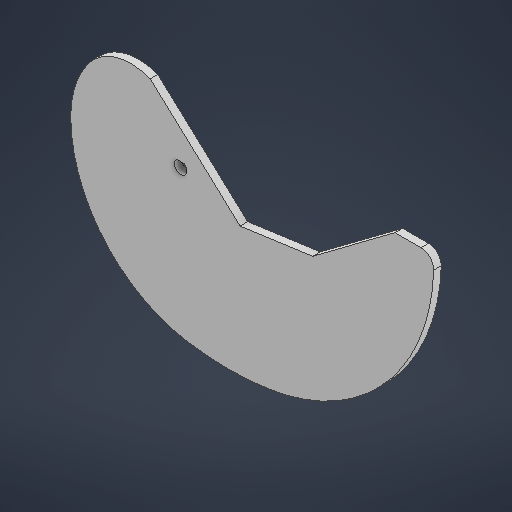
# Autodesk Inventor part: cam3
Saved by Autodesk Inventor 2027 (Build 310192000, 192)
## iProperties
Created: 2026-05-11
Part Number: cam3
Material: Generic
Document SubType Name: Modeling
Designer: alexy
Density: 1 g/cm^3
Appearance: Default
Mass: 17.9661 g
Surface Area: 129.636 cm^2
Volume: 17.9661 cm^3
Author: alexy
Autodesk Inventor part; units mm, degrees
ref_plane "YZ Plane" through (0, 0, 0) normal (1, 0, 0) x (0, 1, 0)
ref_plane "XZ Plane" through (0, 0, 0) normal (0, 1, 0) x (-1, 0, 0)
ref_plane "XY Plane" through (0, 0, 0) normal (0, 0, 1) x (1, 0, 0)
sketch "Sketch1" plane through (0, 0, 0) normal (0, 0, 1) x (1, 0, 0)
  line L0 (0, 0) -> (100, 0)
  arc A0 (100.0128, -3.6299) -> (100, 0) centre (-17.3055, -2.2293) ccw
  arc A1 (35.4459, -78.2987) -> (100.0128, -3.6299) centre (23.4974, -2.7164) ccw
  arc A2 (2.3748, -78.2085) -> (35.4459, -78.2987) centre (19.1908, 24.5253) ccw
  arc A3 (-43.4089, -24.3214) -> (2.3748, -78.2085) centre (11.1953, -24.3214) ccw
  arc A4 (-37.0013, -3.4804) -> (-43.4089, -24.3214) centre (-6.3121, -24.3214) ccw
  line L1 (84.6864, 0) -> (52.1966, -24.3214)
  line L2 (52.1966, -24.3214) -> (23.4974, -28.3171)
  line L3 (23.4974, -28.3171) -> (-12.0135, 4.2661)
  arc A5 (-12.0135, 4.2661) -> (-37.0013, -3.4804) centre (-19.6547, -15.2605) ccw
  point P0 (3.9425, 17.9592)
  dimension "d14" = 100
  constraints: 12 point on circle, 8 end point, 6 centre point, 5 tangent, 1 horizontal, 1 point on line
  measures "d14" distance of L0.start L0.end
extrude "Extrusion1" add sketch "Sketch1" along normal blind 3
sketch "Sketch2" plane through (0, 0, 3) normal (0, 0, 1) x (1, 0, 0)
  arc A0 (-1.5, -18) -> (1.5, -18) centre (0, -20) ccw
  line L0 (-1.5, -18) -> (1.5, -18)
  point P0 (0, 0)
  dimension "d5" = 5
  dimension "d6" = 20
  dimension "d7" = 2
  constraints: 2 end point, 2 point on circle, 1 centre point, 1 horizontal, 1 vertical alignment
  measures "d5" diameter of A0
  measures "d6" distance of point (0, 0) A0.centre
  measures "d7" distance from line of L0 A0.centre
extrude "Extrusion2" cut sketch "Sketch2" against normal blind 3
fillet "Fillet7" radius 5 1 edges at (100, 0, 1.5)
body "Solid1"
